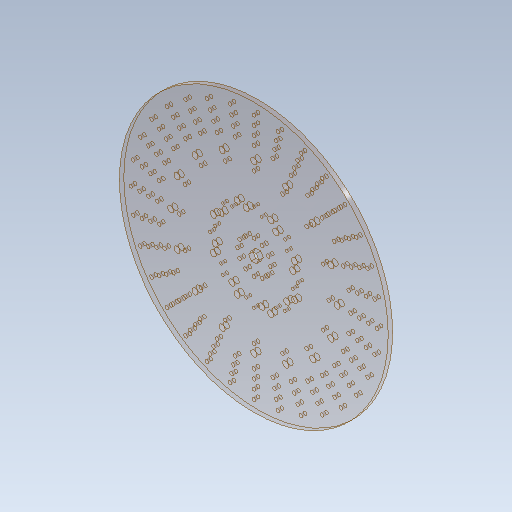
# Autodesk Inventor part: IndexWheelFlatPlatesPolyInside
Saved by Autodesk Inventor 2020 (Build 240168000, 168)
## iProperties
Created: 2020-01-19
Part Number: IndexWheelFlatPlatesPolyInside
Material: Generic
Document SubType Name: Modeling
Designer: srini
Density: 1 g/cm^3
Appearance: Polycarbonate - Smoked
Author: srini
Autodesk Inventor part; units mm, degrees
ref_plane "YZ Plane" through (0, 0, 0) normal (1, 0, 0) x (0, 1, 0)
ref_plane "XZ Plane" through (0, 0, 0) normal (0, 1, 0) x (-1, 0, 0)
ref_plane "XY Plane" through (0, 0, 0) normal (0, 0, 1) x (1, 0, 0)
sketch "Sketch1" plane through (0, 0, 0) normal (0, 0, 1) x (1, 0, 0)
  line L0 (-7.3323, 0) -> (-3.6662, 6.35)
  line L1 (-3.6662, 6.35) -> (3.6662, 6.35)
  line L2 (3.6662, 6.35) -> (7.3323, 0)
  line L3 (7.3323, 0) -> (3.6662, -6.35)
  line L4 (3.6662, -6.35) -> (-3.6662, -6.35)
  line L5 (-3.6662, -6.35) -> (-7.3323, 0)
  circle A0 centre (-31.8143, 47.6135) radius 2.032
  circle A1 centre (-11.1717, -56.164) radius 2.032
  circle A2 centre (-47.6135, 31.8143) radius 4.445
  circle A3 centre (-31.8143, -47.6135) radius 4.445
  circle A4 centre (0, 63.4238) radius 2.032
  circle A5 centre (44.8474, 44.8474) radius 2.032
  circle A6 centre (24.2712, 58.596) radius 4.445
  circle A7 centre (31.8143, 47.6135) radius 4.445
  circle A8 centre (58.596, -24.2712) radius 4.445
  circle A9 centre (31.8143, -47.6135) radius 2.032
  circle A10 centre (63.4238, 0) radius 2.032
  circle A11 centre (-44.8474, 44.8474) radius 2.032
  circle A12 centre (-44.8474, -44.8474) radius 2.032
  circle A13 centre (11.1717, 56.164) radius 2.032
  circle A14 centre (-58.596, 24.2712) radius 4.445
  circle A15 centre (-56.164, 11.1717) radius 2.032
  circle A16 centre (-24.2712, -58.596) radius 4.445
  circle A17 centre (-24.2712, 58.596) radius 4.445
  circle A18 centre (0, -63.4238) radius 2.032
  circle A19 centre (-63.4238, 0) radius 2.032
  circle A20 centre (47.6135, -31.8143) radius 4.445
  circle A21 centre (47.6135, 31.8143) radius 2.032
  circle A22 centre (24.2712, -58.596) radius 4.445
  circle A23 centre (56.164, 11.1717) radius 4.445
  circle A24 centre (58.596, 24.2712) radius 4.445
  circle A25 centre (56.164, -11.1717) radius 2.032
  circle A26 centre (44.8474, -44.8474) radius 2.032
  circle A27 centre (11.1717, -56.164) radius 4.445
  circle A28 centre (-56.164, -11.1717) radius 4.445
  circle A29 centre (-11.1717, 56.164) radius 4.445
  circle A30 centre (-47.6135, -31.8143) radius 2.032
  circle A31 centre (-58.596, -24.2712) radius 4.445
  circle A32 centre (-76.3322, 76.3322) radius 2.5797
  circle A33 centre (-76.3322, -76.3322) radius 2.5797
  circle A34 centre (-107.95, 0) radius 2.5797
  circle A35 centre (-85.043, 85.043) radius 4.445
  circle A36 centre (46.025, 111.1141) radius 4.445
  circle A37 centre (85.043, 85.043) radius 4.445
  circle A38 centre (76.3322, -76.3322) radius 2.5797
  circle A39 centre (120.269, 0) radius 4.445
  circle A40 centre (41.3107, -99.7328) radius 2.5797
  circle A41 centre (99.7328, 41.3107) radius 2.5797
  circle A42 centre (107.95, 0) radius 2.5797
  circle A43 centre (0, 107.95) radius 2.5797
  circle A44 centre (-111.1141, 46.025) radius 4.445
  circle A45 centre (-111.1141, -46.025) radius 4.445
  circle A46 centre (-41.3107, -99.7328) radius 2.5797
  circle A47 centre (0, -120.269) radius 4.445
  circle A48 centre (0, -107.95) radius 2.5797
  circle A49 centre (-85.043, -85.043) radius 4.445
  circle A50 centre (-120.269, 0) radius 4.445
  circle A51 centre (0, 120.269) radius 4.445
  circle A52 centre (76.3322, 76.3322) radius 2.5797
  circle A53 centre (99.7328, -41.3107) radius 2.5797
  circle A54 centre (85.043, -85.043) radius 4.445
  circle A55 centre (46.025, -111.1141) radius 4.445
  circle A56 centre (41.3107, 99.7328) radius 2.5797
  circle A57 centre (111.1141, -46.025) radius 4.445
  circle A58 centre (111.1141, 46.025) radius 4.445
  circle A59 centre (-41.3107, 99.7328) radius 2.5797
  circle A60 centre (-99.7328, 41.3107) radius 2.5797
  circle A61 centre (-99.7328, -41.3107) radius 2.5797
  circle A62 centre (-46.025, -111.1141) radius 4.445
  circle A63 centre (-46.025, 111.1141) radius 4.445
  circle A64 centre (-11.9062, 20.6222) radius 2.5797
  circle A65 centre (20.6222, -11.9063) radius 2.5797
  circle A66 centre (-20.6222, -11.9062) radius 2.5797
  circle A67 centre (-20.6222, 11.9063) radius 2.5797
  circle A68 centre (11.9062, -20.6222) radius 2.5797
  circle A69 centre (20.6222, 11.9062) radius 2.5797
  circle A70 centre (11.9063, 20.6222) radius 2.5797
  circle A71 centre (-23.8125, 0) radius 2.5797
  circle A72 centre (0, -23.8125) radius 2.5797
  circle A73 centre (-11.9063, -20.6222) radius 2.5797
  circle A74 centre (23.8125, 0) radius 2.5797
  circle A75 centre (0, 23.8125) radius 2.5797
  circle A76 centre (0, 0) radius 200.5558
  point P0 (7.3323, 0)
  constraints: 77 centre point, 12 end point
extrude "Extrusion1" add sketch "Sketch1" along normal blind 6.35
sketch "Sketch2" plane through (0, 0, 6.35) normal (0, 0, 1) x (1, 0, 0)
  circle A0 centre (0, 0) radius 200.5558 projected
  circle A1 centre (0, 0) radius 194.2058
  dimension "d2" = 6.35
  constraints: 1 centre point
  measures "d2" radial gap between concentric circles of A0 A1
extrude "Extrusion2" cut sketch "Sketch2" against normal blind 25.4
sketch "Sketch3" plane through (0, 0, 6.35) normal (0, 0, 1) x (1, 0, 0)
  circle A0 centre (0, 139.7) radius 2.5797
  line L0 (0, 0) -> (0, 46.9685) construction
  circle A1 centre (0, 152.4) radius 2.5797
  circle A2 centre (0, 165.1) radius 2.5797
  circle A3 centre (0, 177.8) radius 2.5797
  circle A4 centre (-27.2541, 137.0157) radius 2.5797
  circle A5 centre (-29.7318, 149.4717) radius 2.5797
  circle A6 centre (-32.2094, 161.9276) radius 2.5797
  circle A7 centre (-34.6871, 174.3836) radius 2.5797
  circle A8 centre (-53.4609, 129.066) radius 2.5797
  circle A9 centre (-58.321, 140.7992) radius 2.5797
  circle A10 centre (-63.181, 152.5325) radius 2.5797
  circle A11 centre (-68.0411, 164.2658) radius 2.5797
  circle A12 centre (-77.6132, 116.1563) radius 2.5797
  circle A13 centre (-84.6689, 126.716) radius 2.5797
  circle A14 centre (-91.7246, 137.2756) radius 2.5797
  circle A15 centre (-98.7804, 147.8353) radius 2.5797
  circle A16 centre (-98.7828, 98.7828) radius 2.5797
  circle A17 centre (-107.7631, 107.7631) radius 2.5797
  circle A18 centre (-116.7433, 116.7433) radius 2.5797
  circle A19 centre (-125.7236, 125.7236) radius 2.5797
  circle A20 centre (-116.1563, 77.6132) radius 2.5797
  circle A21 centre (-126.716, 84.6689) radius 2.5797
  circle A22 centre (-137.2756, 91.7246) radius 2.5797
  circle A23 centre (-147.8353, 98.7804) radius 2.5797
  circle A24 centre (-129.066, 53.4609) radius 2.5797
  circle A25 centre (-140.7992, 58.321) radius 2.5797
  circle A26 centre (-152.5325, 63.181) radius 2.5797
  circle A27 centre (-164.2658, 68.0411) radius 2.5797
  circle A28 centre (-137.0157, 27.2541) radius 2.5797
  circle A29 centre (-149.4717, 29.7318) radius 2.5797
  circle A30 centre (-161.9276, 32.2094) radius 2.5797
  circle A31 centre (-174.3836, 34.6871) radius 2.5797
  circle A32 centre (-139.7, 0) radius 2.5797
  circle A33 centre (-152.4, 0) radius 2.5797
  circle A34 centre (-165.1, 0) radius 2.5797
  circle A35 centre (-177.8, 0) radius 2.5797
  circle A36 centre (-137.0157, -27.2541) radius 2.5797
  circle A37 centre (-149.4717, -29.7318) radius 2.5797
  circle A38 centre (-161.9276, -32.2094) radius 2.5797
  circle A39 centre (-174.3836, -34.6871) radius 2.5797
  circle A40 centre (-129.066, -53.4609) radius 2.5797
  circle A41 centre (-140.7992, -58.321) radius 2.5797
  circle A42 centre (-152.5325, -63.181) radius 2.5797
  circle A43 centre (-164.2658, -68.0411) radius 2.5797
  circle A44 centre (-116.1563, -77.6132) radius 2.5797
  circle A45 centre (-126.716, -84.6689) radius 2.5797
  circle A46 centre (-137.2756, -91.7246) radius 2.5797
  circle A47 centre (-147.8353, -98.7804) radius 2.5797
  circle A48 centre (-98.7828, -98.7828) radius 2.5797
  circle A49 centre (-107.7631, -107.7631) radius 2.5797
  circle A50 centre (-116.7433, -116.7433) radius 2.5797
  circle A51 centre (-125.7236, -125.7236) radius 2.5797
  circle A52 centre (-77.6132, -116.1563) radius 2.5797
  circle A53 centre (-84.6689, -126.716) radius 2.5797
  circle A54 centre (-91.7246, -137.2756) radius 2.5797
  circle A55 centre (-98.7804, -147.8353) radius 2.5797
  circle A56 centre (-53.4609, -129.066) radius 2.5797
  circle A57 centre (-58.321, -140.7992) radius 2.5797
  circle A58 centre (-63.181, -152.5325) radius 2.5797
  circle A59 centre (-68.0411, -164.2658) radius 2.5797
  circle A60 centre (-27.2541, -137.0157) radius 2.5797
  circle A61 centre (-29.7318, -149.4717) radius 2.5797
  circle A62 centre (-32.2094, -161.9276) radius 2.5797
  circle A63 centre (-34.6871, -174.3836) radius 2.5797
  circle A64 centre (0, -139.7) radius 2.5797
  circle A65 centre (0, -152.4) radius 2.5797
  circle A66 centre (0, -165.1) radius 2.5797
  circle A67 centre (0, -177.8) radius 2.5797
  circle A68 centre (27.2541, -137.0157) radius 2.5797
  circle A69 centre (29.7318, -149.4717) radius 2.5797
  circle A70 centre (32.2094, -161.9276) radius 2.5797
  circle A71 centre (34.6871, -174.3836) radius 2.5797
  circle A72 centre (53.4609, -129.066) radius 2.5797
  circle A73 centre (58.321, -140.7992) radius 2.5797
  circle A74 centre (63.181, -152.5325) radius 2.5797
  circle A75 centre (68.0411, -164.2658) radius 2.5797
  circle A76 centre (77.6132, -116.1563) radius 2.5797
  circle A77 centre (84.6689, -126.716) radius 2.5797
  circle A78 centre (91.7246, -137.2756) radius 2.5797
  circle A79 centre (98.7804, -147.8353) radius 2.5797
  circle A80 centre (98.7828, -98.7828) radius 2.5797
  circle A81 centre (107.7631, -107.7631) radius 2.5797
  circle A82 centre (116.7433, -116.7433) radius 2.5797
  circle A83 centre (125.7236, -125.7236) radius 2.5797
  circle A84 centre (116.1563, -77.6132) radius 2.5797
  circle A85 centre (126.716, -84.6689) radius 2.5797
  circle A86 centre (137.2756, -91.7246) radius 2.5797
  circle A87 centre (147.8353, -98.7804) radius 2.5797
  circle A88 centre (129.066, -53.4609) radius 2.5797
  circle A89 centre (140.7992, -58.321) radius 2.5797
  circle A90 centre (152.5325, -63.181) radius 2.5797
  circle A91 centre (164.2658, -68.0411) radius 2.5797
  circle A92 centre (137.0157, -27.2541) radius 2.5797
  circle A93 centre (149.4717, -29.7318) radius 2.5797
  circle A94 centre (161.9276, -32.2094) radius 2.5797
  circle A95 centre (174.3836, -34.6871) radius 2.5797
  circle A96 centre (139.7, 0) radius 2.5797
  circle A97 centre (152.4, 0) radius 2.5797
  circle A98 centre (165.1, 0) radius 2.5797
  circle A99 centre (177.8, 0) radius 2.5797
  circle A100 centre (137.0157, 27.2541) radius 2.5797
  circle A101 centre (149.4717, 29.7318) radius 2.5797
  circle A102 centre (161.9276, 32.2094) radius 2.5797
  circle A103 centre (174.3836, 34.6871) radius 2.5797
  circle A104 centre (129.066, 53.4609) radius 2.5797
  circle A105 centre (140.7992, 58.321) radius 2.5797
  circle A106 centre (152.5325, 63.181) radius 2.5797
  circle A107 centre (164.2658, 68.0411) radius 2.5797
  circle A108 centre (116.1563, 77.6132) radius 2.5797
  circle A109 centre (126.716, 84.6689) radius 2.5797
  circle A110 centre (137.2756, 91.7246) radius 2.5797
  circle A111 centre (147.8353, 98.7804) radius 2.5797
  circle A112 centre (98.7828, 98.7828) radius 2.5797
  circle A113 centre (107.7631, 107.7631) radius 2.5797
  circle A114 centre (116.7433, 116.7433) radius 2.5797
  circle A115 centre (125.7236, 125.7236) radius 2.5797
  circle A116 centre (77.6132, 116.1563) radius 2.5797
  circle A117 centre (84.6689, 126.716) radius 2.5797
  circle A118 centre (91.7246, 137.2756) radius 2.5797
  circle A119 centre (98.7804, 147.8353) radius 2.5797
  circle A120 centre (53.4609, 129.066) radius 2.5797
  circle A121 centre (58.321, 140.7992) radius 2.5797
  circle A122 centre (63.181, 152.5325) radius 2.5797
  circle A123 centre (68.0411, 164.2658) radius 2.5797
  circle A124 centre (27.2541, 137.0157) radius 2.5797
  circle A125 centre (29.7318, 149.4717) radius 2.5797
  circle A126 centre (32.2094, 161.9276) radius 2.5797
  circle A127 centre (34.6871, 174.3836) radius 2.5797
  dimension "d5" = 5.1594
  dimension "d6" = 139.7
  dimension "d9" = 12.7
  dimension "d16" = 360
  constraints: 128 centre point, 2 end point, 2 vertical, 1 vertical alignment, 263 other
  measures "d5" diameter of A0
  measures "d6" distance of L0.start A0.centre
  measures "d9" distance of A0.centre A1.centre
extrude "Extrusion3" cut sketch "Sketch3" against normal blind 25.4
body "Solid1"
